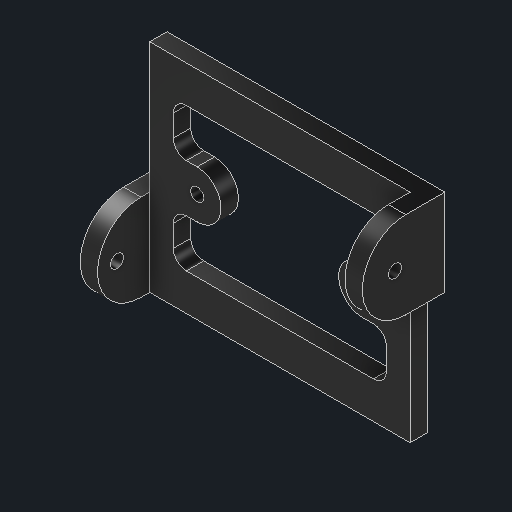
# Autodesk Inventor part: LED_mount
Saved by Autodesk Inventor 2026.1 (Build 301233000, 233)
## iProperties
Created: 2026-01-20
Part Number: LED_mount
Material: ABS Plastic
Document SubType Name: Modeling
Designer: aleja
Density: 1.06 g/cm^3
Appearance: Glossy - Black
Author: aleja
Autodesk Inventor part; units mm, degrees
ref_plane "YZ Plane" through (0, 0, 0) normal (1, 0, 0) x (0, 1, 0)
ref_plane "XZ Plane" through (0, 0, 0) normal (0, 1, 0) x (-1, 0, 0)
ref_plane "XY Plane" through (0, 0, 0) normal (0, 0, 1) x (1, 0, 0)
sketch "Sketch1" plane through (0, 0, 0) normal (0, 1, 0) x (-1, 0, 0)
  line L0 (-30, 25) -> (30, 25)
  line L1 (30, 25) -> (30, -25)
  line L2 (30, -25) -> (-30, -25)
  line L3 (-30, -25) -> (-30, 25)
  line L4 (-30, 25) -> (30, -25) construction
  line L5 (30, 25) -> (-30, -25) construction
  point P0 (0, 0)
  dimension "d0" = 60
  dimension "d1" = 50
  constraints: 12 end point, 2 midpoint, 2 parallel, 1 horizontal, 1 perpendicular
  measures "d0" distance of L1.end L2.end
  measures "d1" distance of L0.end L1.end
extrude "Extrusion1" add sketch "Sketch1" along normal blind 4
sketch "Sketch2" plane through (0, 4, 0) normal (0, 1, 0) x (1, 0, 0)
  line L0 (24.55, -16.5) -> (-24.55, -16.5)
  line L1 (-24.55, -16.5) -> (-24.55, 16.5)
  line L2 (-24.55, 16.5) -> (24.55, 16.5)
  line L3 (24.55, 16.5) -> (24.55, -16.5)
  line L4 (24.55, -16.5) -> (-24.55, 16.5) construction
  line L5 (-24.55, -16.5) -> (24.55, 16.5) construction
  line L6 (-24.55, 0) -> (-19.05, 0) construction
  arc A0 (-19.05, -5.5) -> (-19.05, 5.5) centre (-19.05, 0) ccw
  circle A1 centre (-19.05, 0) radius 1.5
  line L7 (-24.55, -5.5) -> (-19.05, -5.5)
  line L8 (-19.05, 5.5) -> (-24.55, 5.5)
  line L9 (0, 0) -> (0, 7.8655) construction
  arc A2 (19.05, 5.5) -> (19.05, -5.5) centre (19.05, 0) ccw
  circle A3 centre (19.05, 0) radius 1.5
  line L10 (24.55, -5.5) -> (19.05, -5.5)
  line L11 (19.05, 5.5) -> (24.55, 5.5)
  point P0 (0, 0)
  dimension "d4" = 49.1
  dimension "d5" = 33
  dimension "d6" = 5.5
  dimension "d7" = 3
  constraints: 24 end point, 6 symmetric about line, 4 centre point, 4 midpoint, 4 parallel, 4 point on circle, 3 coincident, 2 horizontal, 2 perpendicular, 2 point on line, 1 tangent, 1 vertical, 2 other
  measures "d4" distance of L1.end L2.end
  measures "d5" distance of L0.end L1.end
  measures "d6" distance of L6.start L6.end
  measures "d7" diameter of A1
extrude "Extrusion2" cut sketch "Sketch2" against normal through all contours L0 L1 L7 A0 L8 L2 L3 L11 A2 L10 | A1 | A3
sketch "Sketch3" plane through (0, 0, 0) normal (0, -1, 0) x (1, 0, 0)
  line L0 (-30, 25) -> (30, 25) projected
  line L1 (-30, 25) -> (-34, 25)
  line L2 (-34, 25) -> (-34, 5)
  line L3 (-34, 5) -> (-30, 5)
  line L4 (-30, 5) -> (-30, 25)
  line L5 (-34, 25) -> (-10, 25)
  line L6 (-10, 25) -> (-10, 29)
  line L7 (-10, 29) -> (-34, 29)
  line L8 (-34, 29) -> (-34, 25)
  line L9 (-30, -25) -> (-30, 25) projected
  line L10 (-30, 0) -> (-43.5069, 0) construction
  line L11 (-30, -25) -> (-34, -25)
  line L12 (-34, -25) -> (-34, -5)
  line L13 (-34, -5) -> (-30, -5)
  line L14 (-30, -5) -> (-30, -25)
  line L15 (-34, -25) -> (-10, -25)
  line L16 (-10, -25) -> (-10, -29)
  line L17 (-10, -29) -> (-34, -29)
  line L18 (-34, -29) -> (-34, -25)
  line L19 (0, 25) -> (0, 63.1817) construction
  line L20 (30, 25) -> (34, 25)
  line L21 (34, 25) -> (34, 5)
  line L22 (34, 5) -> (30, 5)
  line L23 (30, 5) -> (30, 25)
  line L24 (34, 25) -> (10, 25)
  line L25 (10, 25) -> (10, 29)
  line L26 (10, 29) -> (34, 29)
  line L27 (34, 29) -> (34, 25)
  line L28 (30, -25) -> (30, 25)
  line L29 (30, 0) -> (43.5069, 0) construction
  line L30 (30, -25) -> (34, -25)
  line L31 (34, -25) -> (34, -5)
  line L32 (34, -5) -> (30, -5)
  line L33 (30, -5) -> (30, -25)
  line L34 (34, -25) -> (10, -25)
  line L35 (10, -25) -> (10, -29)
  line L36 (10, -29) -> (34, -29)
  line L37 (34, -29) -> (34, -25)
  line L38 (30, -25) -> (30, -29)
  line L39 (30, 25) -> (30, 29)
  point P0 (0, 0)
  point P1 (-30, -25)
  point P2 (-30, -5)
  point P3 (30, -5)
  point P4 (30, -25)
  point P5 (30, -25)
  dimension "d21" = 4
  dimension "d22" = 20
  dimension "d23" = 24
  dimension "d24" = 4
  constraints: 76 end point, 21 symmetric about line, 4 parallel, 3 horizontal, 3 perpendicular, 3 point on line, 2 midpoint, 1 vertical
  measures "d21" distance of L3.end L2.end
  measures "d22" distance of L2.end L1.end
  measures "d23" distance of L7.end L6.end
  measures "d24" distance of L6.end L5.end
extrude "Extrusion3" add sketch "Sketch3" along normal blind 15 and the other way blind 4 contours L20 L21 L22 L23 | L11 L12 L13 L9
fillet "Fillet1" radius 3 12 edges at (24.55, 2, -16.5) (24.55, 2, -5.5) (24.55, 2, 16.5) (24.55, 2, 5.5) (-24.55, 2, -16.5) (-24.55, 2, -5.5) (-24.55, 2, 5.5) (-24.55, 2, 16.5) (19.05, 2, 5.5) (19.05, 2, -5.5) (-19.05, 2, -5.5) (-19.05, 2, 5.5)
sketch "Sketch7" plane through (-30, 0, -5) normal (1, 0, 0) x (0, 0, -1)
  line L0 (0, -15) -> (20, -15) projected
  line L1 (10, -15) -> (10, 0)
  line L2 (20, 0) -> (0, 0) projected
  circle A0 centre (10, -7.5) radius 1.5
  line L3 (-5, 0) -> (-5, -12.3055)
  circle A1 centre (-20, -7.5) radius 1.5
  dimension "d47" = 3
  constraints: 4 end point, 3 midpoint, 2 centre point, 1 symmetric about line, 1 vertical, 1 other
  measures "d47" diameter of A0
extrude "Extrusion8" cut sketch "Sketch7" along normal through all both and the other way through all
sketch "Sketch9" plane through (0, -15, 0) normal (0, -1, 0) x (1, 0, 0)
  line L0 (-34, -5) -> (-34, -25) projected
  line L1 (-30, -25) -> (-30, -5) projected
  line L2 (-30, -5) -> (-34, -5) projected
  line L3 (-34, -25) -> (-30, -25) projected
  line L4 (-34, 5) -> (-30, 5) projected
  line L5 (-30, 5) -> (-30, 25) projected
  line L6 (-30, 25) -> (-34, 25) projected
  line L7 (-34, 25) -> (-34, 5) projected
  line L8 (30, 29) -> (10, 29) projected
  line L9 (10, 29) -> (10, 25) projected
  line L10 (10, 25) -> (30, 25) projected
  line L11 (30, 25) -> (30, 29) projected
  line L12 (10, -29) -> (30, -29) projected
  line L13 (30, -29) -> (30, -25) projected
  line L14 (30, -25) -> (10, -25) projected
  line L15 (10, -25) -> (10, -29) projected
  point P0 (0, 0)
extrude "Extrusion10" cut sketch "Sketch9" against normal blind 3
fillet "Fillet2" radius 10 4 edges at (-32, -12, -5) (-32, -12, -25) (32, -15, 5) (32, -15, 25)
body "Solid1"
